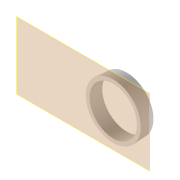
# Autodesk Inventor part: 10_Filteslide_25mm_insert
Saved by Autodesk Inventor 2022.5 (Build 265521000, 521)
## iProperties
Created: 2023-11-21
Part Number: 10_Filteslide_25mm_insert
Material: Generisch
Document SubType Name: Modeling
Designer: diederichbenedict
Density: 1 g/cm^3
Appearance: Vorgabe
Author: diederichbenedict
Autodesk Inventor part; units mm, degrees
ref_plane "YZ Plane" through (0, 0, 0) normal (1, 0, 0) x (0, 1, 0)
ref_plane "XZ Plane" through (0, 0, 0) normal (0, 1, 0) x (-1, 0, 0)
ref_plane "Arbeitsebene1" through (0, 0, 0) normal (0, 0, 1) x (1, 0, 0)
sketch "Skizze1" plane through (0, 0, 0) normal (0, 0, 1) x (1, 0, 0)
  circle A0 centre (18.229, 0) radius 12.775 projected
  arc A1 (-21.8552, 14.25) -> (-23.8552, 12.25) centre (-21.8552, 12.25) ccw projected
  line L0 (-23.8552, 12.25) -> (-23.8552, -12.25) projected
  arc A2 (-23.8552, -12.25) -> (-21.8552, -14.25) centre (-21.8552, -12.25) ccw projected
  line L1 (-21.8552, -14.25) -> (18.229, -14.25) projected
  arc A3 (18.229, -14.25) -> (18.229, 14.25) centre (18.229, 0) ccw projected
  line L2 (18.229, 14.25) -> (-21.8552, 14.25) projected
  circle A4 centre (18.229, 0) radius 11
  point P0 (0, 0)
  dimension "d0" = 22
  constraints: 1 centre point, 1 coincident
  measures "d0" diameter of A4
ref_plane "Arbeitsebene2" through (5.454, -12.775, -6.25) normal (0, 0, 1) x (1, 0, 0)
extrude "Extrusion1" add sketch "Skizze1" against normal up to surface (6.25 mm away) draft -3 contours A0
